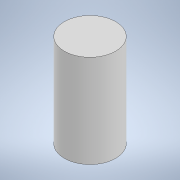
# Autodesk Inventor part: obiektyw1
Saved by Autodesk Inventor 2020 (Build 240168000, 168)
## iProperties
Created: 2019-12-30
Part Number: obiektyw1
Material: Ogólny
Document SubType Name: Modeling
Designer: macie
Density: 1 g/cm^3
Appearance: Domyślna
Author: macie
Autodesk Inventor part; units mm, degrees
ref_plane "YZ Plane" through (0, 0, 0) normal (1, 0, 0) x (0, 1, 0)
ref_plane "XZ Plane" through (0, 0, 0) normal (0, 1, 0) x (-1, 0, 0)
ref_plane "XY Plane" through (0, 0, 0) normal (0, 0, 1) x (1, 0, 0)
sketch "Szkic1" plane through (0, 0, 0) normal (0, 0, 1) x (1, 0, 0)
  line L0 (0, 0) -> (14.1, 0) construction
  line L1 (0, 0) -> (0, -32.7) construction
  line L2 (14.1, 0) -> (14.1, -32.7)
  line L3 (0, 0) -> (0, 3)
  arc A0 (9.0253, 0) -> (0, 3) centre (-0.3652, -13.1746) ccw
  line L4 (9.0253, 0) -> (14.1, 1.8667)
  line L5 (14.1, 1.8667) -> (14.1, 0)
  line L6 (0, 0) -> (0, -32.7)
  line L7 (14.1, -32.7) -> (0, -32.7)
  line L8 (9.0253, 0) -> (9.0253, -32.7)
  line L9 (0, 0) -> (9.0253, 0)
  dimension "d0" = 14.1
  dimension "d1" = 32.7
  dimension "d2" = 3
  constraints: 20 end point, 4 vertical, 2 perpendicular, 2 point on circle, 2 point on line, 1 centre point, 1 collinear, 1 horizontal
  measures "d0" distance of L0.start L0.end
  measures "d1" distance of L0.start L1.end
  measures "d2" distance of L0.start L3.end
revolve "Obrót2" add sketch "Szkic1" angle 360 about axis through (0, 0, 0) along (0, -1, 0) contours L7 L6 L9 L8
